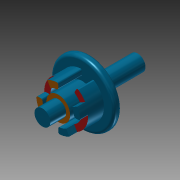
# Autodesk Inventor part: Spool Main Section Mk1
Saved by Autodesk Inventor 2015 (Build 190159000, 159)
## iProperties
Created: 2016-11-23
Part Number: Spool Main Section Mk1
Material: Generic
Document SubType Name: Modeling
Designer: Markus
Density: 1 g/cm^3
Appearance: Sky Blue Dark
Author: Markus
Autodesk Inventor part; units mm, degrees
ref_plane "YZ Plane" through (0, 0, 0) normal (1, 0, 0) x (0, 1, 0)
ref_plane "XZ Plane" through (0, 0, 0) normal (0, 1, 0) x (-1, 0, 0)
ref_plane "XY Plane" through (0, 0, 0) normal (0, 0, 1) x (1, 0, 0)
sketch "Sketch1" plane through (0, 0, 0) normal (0, 0, 1) x (1, 0, 0)
  circle A0 centre (0, 0) radius 25.4
  circle A1 centre (0, 0) radius 6.35
  dimension "d0" = 50.8
  dimension "d4" = 12.7
  constraints: 2 centre point, 2 coincident
  measures "d0" diameter of A0
  measures "d4" diameter of A1
extrude "Extrusion1" add sketch "Sketch1" along normal blind 6.35
sketch "Sketch2" plane through (0, 0, 6.35) normal (0, 0, 1) x (1, 0, 0)
  circle A0 centre (0, 0) radius 25.4 construction
  circle A1 centre (0, 0) radius 9.525
  circle A2 centre (0, 0) radius 6.35
  line L0 (0, 0) -> (0, 17.5641) construction
  line L1 (0, 0) -> (0, -17.5641) construction
  line L2 (0, 17.5641) -> (0, 12.7)
  line L3 (0, 0) -> (8.7821, 15.211) construction
  line L4 (8.7821, 15.211) -> (6.35, 10.9985)
  line L5 (0, 0) -> (-8.782, -15.211) construction
  line L6 (0, -12.7) -> (0, -17.5641)
  line L7 (-8.782, -15.211) -> (-6.35, -10.9985)
  arc A3 (0, 12.7) -> (-6.35, -10.9985) centre (0, 0) ccw
  arc A4 (0, -12.7) -> (6.35, 10.9985) centre (0, 0) ccw
  arc A5 (0, 17.5641) -> (-8.782, -15.211) centre (0, 0) ccw
  arc A6 (0, -17.5641) -> (8.7821, 15.211) centre (0, 0) ccw
  dimension "d5" = 19.05
  dimension "d6" = 12.7
  dimension "d8" = 30
  dimension "d9" = 30
  dimension "d10" = 12.7
  dimension "d11" = 17.5641
  dimension "d12" = 17.5641
  dimension "d13" = 12.7
  constraints: 16 end point, 8 point on circle, 6 centre point, 5 point on line, 4 coincident, 1 collinear, 1 vertical
  measures "d5" diameter of A1
  measures "d6" diameter of A2
  measures "d8" angle of L0 L3
  measures "d9" angle of L1 L5
  measures "d10" radius of A3
  measures "d11" radius of A5
  measures "d12" radius of A6
  measures "d13" radius of A4
extrude "Extrusion2" add sketch "Sketch2" along normal blind 12.7
fillet "Fillet1" radius 1.27 8 edges at (0, 17.5641, 12.7) (0, 12.7, 12.7) (8.7821, 15.211, 12.7) (6.35, 10.9985, 12.7) (0, -12.7, 12.7) (0, -17.5641, 12.7) (-8.782, -15.211, 12.7) (-6.35, -10.9985, 12.7)
sketch "Sketch3" plane through (0, 0, 19.05) normal (0, 0, 1) x (1, 0, 0)
  circle A0 centre (0, 0) radius 6.35 projected
  circle A1 centre (0, 0) radius 9.525 projected
extrude "Extrusion3" add sketch "Sketch3" along normal blind 6.35
sketch "Sketch4" plane through (0, 0, 19.05) normal (0, 0, 1) x (1, 0, 0)
  arc A0 (-1.1545, 12.6474) -> (-7.3236, -10.3757) centre (0, 0) ccw projected
  line L0 (-8.1223, -14.0682) -> (-6.9561, -12.0483) projected
  arc A1 (-1.369, 17.5107) -> (-9.9409, -14.4802) centre (0, 0) ccw projected
  circle A2 centre (0, 0) radius 25.4 construction
  line L1 (0, 25.4) -> (0, -25.4) construction
  line L2 (0, 0) -> (-8.782, 15.211) construction
  line L3 (0, 0) -> (8.782, -15.211) construction
  arc A3 (-6.9561, -12.0483) -> (-7.3236, -10.3757) centre (-8.0559, -11.4133) ccw projected
  arc A4 (-1.1545, 12.6474) -> (-7.3236, -10.3757) centre (0, 0) ccw projected
  arc A5 (-1.1545, 12.6474) -> (0, 13.9122) centre (-1.27, 13.9122) ccw projected
  line L4 (0, 13.9122) -> (0, 16.2445) projected
  arc A6 (0, 16.2445) -> (-1.369, 17.5107) centre (-1.27, 16.2445) ccw projected
  arc A7 (-1.369, 17.5107) -> (-9.9409, -14.4802) centre (0, 0) ccw projected
  arc A8 (-9.9409, -14.4802) -> (-8.1223, -14.0682) centre (-9.2221, -13.4332) ccw projected
  line L5 (-8.1223, -14.0682) -> (-6.9561, -12.0483) projected
  line L6 (-8.782, 15.211) -> (-6.35, 10.9985)
  arc A9 (0, -16.2445) -> (1.369, -17.5107) centre (1.27, -16.2445) ccw projected
  arc A10 (1.369, -17.5107) -> (9.9409, 14.4802) centre (0, 0) ccw projected
  arc A11 (9.9409, 14.4802) -> (8.1223, 14.0682) centre (9.2221, 13.4332) ccw projected
  line L7 (8.1223, 14.0682) -> (6.9561, 12.0483) projected
  arc A12 (6.9561, 12.0483) -> (7.3236, 10.3757) centre (8.0559, 11.4133) ccw projected
  arc A13 (1.1545, -12.6474) -> (7.3236, 10.3757) centre (0, 0) ccw projected
  arc A14 (1.1545, -12.6474) -> (0, -13.9122) centre (1.27, -13.9122) ccw projected
  line L8 (0, -13.9122) -> (0, -16.2445) projected
  line L9 (6.35, -10.9985) -> (8.782, -15.211)
  arc A15 (-1.369, 17.5107) -> (-8.782, 15.211) centre (0, 0) ccw
  arc A16 (-1.1545, 12.6474) -> (-6.35, 10.9985) centre (0, 0) ccw
  arc A17 (-1.1545, 12.6474) -> (0, 13.9122) centre (-1.27, 13.9122) ccw
  arc A18 (0, 16.2445) -> (-1.369, 17.5107) centre (-1.27, 16.2445) ccw
  line L10 (0, 16.2445) -> (0, 13.9122)
  dimension "d19" = 30
  dimension "d20" = 12.7
  constraints: 13 point on circle, 12 end point, 4 centre point, 4 coincident, 3 collinear, 2 point on line, 2 vertical, 1 midpoint
  measures "d19" angle of L1 L2
  measures "d20" radius of A16
extrude "Extrusion4" add sketch "Sketch4" along normal blind 6.35 contours A0 L6 A1 A6 L4 A5
pattern_circular "Circular Pattern1" count 4 over 360 about axis through (0, 0, 0) along (0, 0, 1) of "Extrusion4"
sketch "Sketch5" plane through (0, 0, 0) normal (0, 0, -1) x (-1, 0, 0)
  circle A0 centre (0, 0) radius 6.35
  circle A1 centre (0, 0) radius 6.35 projected
  constraints: 1 centre point, 1 coincident, 1 concentric
extrude "Extrusion5" add sketch "Sketch5" along normal blind 38.1 and the other way blind 38.1
fillet "Fillet2" radius 2.54 2 edges at (-25.4, 0, 6.35) (-25.4, 0, 0)
equation "\"d12\" = d11"
equation "\"d13\" = d10"
body "Solid1"
